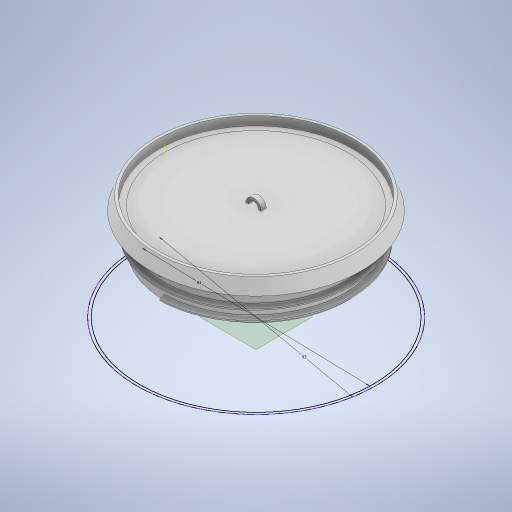
# Autodesk Inventor part: 탄두2
Saved by Autodesk Inventor 2023 (Build 270158000, 158)
## iProperties
Created: 2023-10-03
Part Number: 탄두2
Material: 일반
Document SubType Name: Modeling
Designer: rlatk
Density: 1 g/cm^3
Appearance: 기본값
Author: rlatk
Autodesk Inventor part; units mm, degrees
ref_plane "YZ Plane" through (0, 0, 0) normal (1, 0, 0) x (0, 1, 0)
ref_plane "XZ Plane" through (0, 0, 0) normal (0, 1, 0) x (-1, 0, 0)
ref_plane "XY Plane" through (0, 0, 0) normal (0, 0, 1) x (1, 0, 0)
sketch "스케치1" plane through (0, 0, 0) normal (0, 1, 0) x (-1, 0, 0)
  circle A0 centre (0, 0) radius 46.5
  dimension "d0" = 93
  constraints: 1 centre point, 1 coincident
  measures "d0" diameter of A0
sketch "스케치2" plane through (0, 0, 0) normal (0, 0, 1) x (1, 0, 0)
  line L0 (46.5, 0) -> (-46.5, 0) projected
  line L1 (0, 0) -> (0, 90)
  arc A0 (0, 90) -> (-46.5, 0) centre (59.9038, 2.0372) ccw
  line L2 (-20.2736, 0) -> (-20.2736, 36)
  arc A1 (0, 87.7361) -> (-42.8811, 0) centre (62.0049, 3.084) ccw
  line L3 (0, -19.1775) -> (0, 115.0652) projected
  line L4 (-43.0533, 36) -> (0, 36)
  line L5 (-40.9547, 36) -> (-37.6316, 36)
  line L6 (-37.6316, 36) -> (-37.6316, 23.2038)
  line L7 (-37.6316, 23.2038) -> (-40.9547, 23.2038)
  line L8 (-40.9547, 23.2038) -> (-40.9547, 36)
  line L9 (-35.5316, 36) -> (0, 36)
  line L10 (0, 36) -> (0, 23.2038)
  line L11 (0, 23.2038) -> (-35.5316, 23.2038)
  line L12 (-35.5316, 23.2038) -> (-35.5316, 36)
  line L13 (-40.349, 37.7484) -> (-35.5316, 37.7484)
  line L14 (-35.5316, 37.7484) -> (-35.5316, 36)
  line L15 (-40.349, 37.7484) -> (0, 37.7484)
  line L16 (0, 37.7484) -> (0, 23.2038)
  line L17 (0, 41.2482) -> (0, 23.2038)
  line L18 (-29.8738, 59.1853) -> (0, 59.1853)
  line L19 (-29.8738, 59.1853) -> (-26.6903, 59.1853)
  line L20 (-26.6903, 59.1853) -> (-26.6903, 53.7544)
  line L21 (-26.6903, 53.7544) -> (-29.8738, 53.7544)
  line L22 (-29.8738, 53.7544) -> (-29.8738, 59.1853)
  line L23 (-26.6903, 53.7544) -> (-26.6903, 37.7484)
  line L24 (-32.2689, 36) -> (-32.2689, 23.2038)
  line L25 (-39.0326, 41.2482) -> (-35.7401, 41.2482)
  line L26 (-35.7401, 41.2482) -> (-35.7401, 37.7484)
  point P0 (-43.0533, 28.9768)
  point P1 (-40.9547, 23.3299)
  point P2 (-39.0326, 41.2482)
  point P3 (-37.0353, 37.7484)
  point P4 (-37.63, 36)
  point P5 (-29.8738, 53.7682)
  dimension "d1" = 90
  dimension "d2" = 36
  dimension "d36" = 2.1
  dimension "d37" = 1.7485
  constraints: 50 end point, 13 point on line, 11 point on circle, 10 perpendicular, 6 parallel, 5 horizontal, 2 centre point, 2 collinear, 1 vertical
  measures "d1" distance of L1.start L1.end
  measures "d2" distance of L2.start L2.end
  measures "d36" distance between parallel lines of L6 L12
  measures "d37" distance between parallel lines of L4 L15
ref_plane "작업 평면2" through (0, 0, 0) normal (0, -1, 0) x (1, 0, 0)
sketch "스케치3" plane through (0, 0, 0) normal (0, -1, 0) x (1, 0, 0)
  circle A0 centre (0, 0) radius 45.5
  circle A1 centre (0, 0) radius 46.5
  dimension "d6" = 91
  constraints: 2 centre point, 2 coincident
  measures "d6" diameter of A0
ref_plane "작업 평면1" through (0, 36, 0) normal (0, 1, 0) x (1, 0, 0)
sketch "스케치5" plane through (0, 36, 0) normal (0, 1, 0) x (1, 0, 0)
  point P0 (0, 0)
sketch "스케치8" plane through (0, 0, 0) normal (1, 0, 0) x (0, 1, 0)
  line L0 (23.2038, 35.5316) -> (36, 35.5316) projected
  line L1 (23.8038, 35.5316) -> (25.3038, 35.5316)
  line L2 (25.3038, 35.5316) -> (25.3038, 37.5316)
  line L3 (25.3038, 37.5316) -> (23.8038, 37.5316)
  line L4 (23.8038, 37.5316) -> (23.8038, 35.5316)
  line L5 (23.2038, -35.5316) -> (23.2038, 35.5316) projected
  line L6 (23.2038, 35.5316) -> (23.2038, 38.5251)
  line L7 (25.3038, 35.5316) -> (24.8038, 37.5316)
  line L8 (24.3038, 37.5316) -> (23.8038, 35.5316)
  point P0 (0, 0)
  dimension "d40" = 1.5
  dimension "d41" = 2
  dimension "d42" = 0.6
  dimension "d43" = 0.5
  dimension "d44" = 0.5
  constraints: 14 end point, 3 point on line, 2 parallel, 1 horizontal, 1 perpendicular, 1 vertical
  measures "d40" distance of L3.end L2.end
  measures "d41" distance of L2.end L1.end
  measures "d42" distance between parallel lines of L6 L4
  measures "d43" distance of L3.end L8.start
  measures "d44" distance of L7.end L2.end
coil "코일3" sketch "스케치8" operation add axis through (0, -10, 0) along (0, 1, 0) pitch 4 turns 2 hand right contours L8 L3 L7 L0
revolve "회전4" add sketch "스케치2" angle 360 about axis through (0, -10, 0) along (0, 1, 0) contours L4 L14 L15 L1 | L11 L12 L4 L24 | A0 L13 A1 L4 | A1 L13 L14 L4 | A0 L25 A1 L13 | A1 L26 L13
sketch "스케치11" plane through (0, 0, 0) normal (0, 0, 1) x (1, 0, 0)
  line L0 (37.0353, 37.7484) -> (-37.0353, 37.7484) projected
  circle A0 centre (0, 37.7484) radius 3
  circle A1 centre (0, 37.7484) radius 2
  point P0 (0, 0)
  point P1 (-2, 37.7484)
  point P2 (2, 37.7484)
  point P3 (3, 37.7484)
  point P4 (-3, 37.7484)
  dimension "d60" = 6
  dimension "d61" = 4
  constraints: 2 centre point, 1 coincident, 1 midpoint
  measures "d60" diameter of A0
  measures "d61" diameter of A1
extrude "돌출4" add sketch "스케치11" along normal blind 1 and the other way blind 1 contours L0 A1 A0 picked at (2.4467, 38.7623)
sketch "스케치12" plane through (0, 41.2482, 0) normal (0, 1, 0) x (1, 0, 0)
  circle A0 centre (0, 0) radius 39.0326 projected
  circle A1 centre (0, 0) radius 35.7401 projected
  circle A2 centre (0, 0) radius 39.0326
  circle A3 centre (0, 0) radius 35.7401
  circle A4 centre (0, 0) radius 38
  dimension "d66" = 76
  constraints: 3 centre point, 3 coincident, 2 concentric
  measures "d66" diameter of A4
sketch "스케치13" plane through (0, 0, 0) normal (0, 0, 1) x (1, 0, 0)
  line L0 (-35.7401, 41.2482) -> (-35.7401, 37.7484) projected
  point P0 (0, 0)
extrude "돌출5" cut sketch "스케치12" against normal blind 3.5 contours A4
